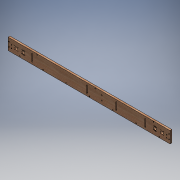
# Autodesk Inventor part: licht_150_top
Saved by Autodesk Inventor 2016 SP2 (Build 200236200, 236)
## iProperties
Created: 2018-01-11
Part Number: licht_150_top
Material: Spanplatte
Document SubType Name: Blech
Designer: schueler
Density: 1 g/cm^3
Sheet Metal Rule: Standard_mm
Appearance: Birke - natur- poliert
Mass: 2150.35 g
Surface Area: 3364.44 cm^2
Volume: 2150.35 cm^3
Author: schueler
Autodesk Inventor part; units mm, degrees
ref_plane "YZ Plane" through (0, 0, 0) normal (1, 0, 0) x (0, 1, 0)
ref_plane "XZ Plane" through (0, 0, 0) normal (0, 1, 0) x (-1, 0, 0)
ref_plane "XY Plane" through (0, 0, 0) normal (0, 0, 1) x (1, 0, 0)
sketch "Skizze1" plane through (0, 0, 0) normal (0, 1, 0) x (-1, 0, 0)
  line L0 (0, 0) -> (1392, 0)
  line L1 (1392, 0) -> (1392, -100)
  line L2 (1392, -100) -> (0, -100)
  line L3 (462, 0) -> (462, -100) construction
  line L4 (712, 0) -> (712, -100) construction
  line L5 (1292, 0) -> (1292, -100) construction
  line L6 (0, -92) -> (1392, -92) construction
  circle A0 centre (1292, -92) radius 1.5
  line L7 (1384, 0) -> (1384, -100) construction
  circle A1 centre (1384, -70) radius 1.5
  circle A2 centre (1384, -30) radius 1.5
  line L8 (1184.5, -137) -> (1184.5, -21) construction
  line L9 (1392, -8) -> (0, -8) construction
  circle A3 centre (1142, -8) radius 1.5
  line L10 (212, 0) -> (212, -100) construction
  line L11 (1092, 0) -> (1092, -100) construction
  line L12 (892, 0) -> (892, -100) construction
  line L13 (692, 0) -> (692, -100) construction
  line L14 (212, -16) -> (212, -16)
  line L15 (207, -21) -> (207, -79)
  line L16 (212, -84) -> (212, -84)
  line L17 (217, -79) -> (217, -21)
  arc A4 (217, -21) -> (212, -16) centre (212, -21) ccw
  arc A5 (212, -16) -> (207, -21) centre (212, -21) ccw
  arc A6 (207, -79) -> (212, -84) centre (212, -79) ccw
  arc A7 (212, -84) -> (217, -79) centre (212, -79) ccw
  circle A8 centre (1092, -92) radius 1.5
  circle A9 centre (892, -92) radius 1.5
  line L18 (92, 0) -> (92, -100) construction
  circle A10 centre (142, -8) radius 1.5
  circle A11 centre (92, -92) radius 1.5
  circle A12 centre (692, -92) radius 1.5
  circle A13 centre (642, -8) radius 1.5
  line L19 (292, 0) -> (292, -100) construction
  line L20 (492, 0) -> (492, -100) construction
  circle A14 centre (292, -92) radius 1.5
  circle A15 centre (492, -92) radius 1.5
  line L21 (462, -16) -> (462, -16)
  line L22 (457, -21) -> (457, -79)
  line L23 (467, -79) -> (467, -21)
  line L24 (1184.5, -84) -> (212, -84) construction
  line L25 (212, -16) -> (1184.5, -16) construction
  line L26 (1184.5, -21) -> (212, -21) construction
  line L27 (212, -79) -> (1184.5, -79) construction
  line L28 (712, -16) -> (712, -16)
  line L29 (707, -21) -> (707, -79)
  line L30 (712, -84) -> (712, -84)
  line L31 (717, -79) -> (717, -21)
  line L32 (1184.5, -16) -> (1184.5, -16)
  line L33 (1189.5, -21) -> (1189.5, -79)
  line L34 (1184.5, -84) -> (1184.5, -84)
  line L35 (1179.5, -79) -> (1179.5, -21)
  arc A16 (1189.5, -21) -> (1184.5, -16) centre (1184.5, -21) ccw
  arc A17 (1184.5, -16) -> (1179.5, -21) centre (1184.5, -21) ccw
  arc A18 (1179.5, -79) -> (1184.5, -84) centre (1184.5, -79) ccw
  arc A19 (1184.5, -84) -> (1189.5, -79) centre (1184.5, -79) ccw
  arc A20 (707, -79) -> (712, -84) centre (712, -79) ccw
  arc A21 (712, -84) -> (717, -79) centre (712, -79) ccw
  arc A22 (717, -21) -> (712, -16) centre (712, -21) ccw
  arc A23 (712, -16) -> (707, -21) centre (712, -21) ccw
  arc A24 (467, -21) -> (462, -16) centre (462, -21) ccw
  arc A25 (462, -16) -> (457, -21) centre (462, -21) ccw
  arc A26 (457, -79) -> (462, -84) centre (462, -79) ccw
  arc A27 (462, -84) -> (467, -79) centre (462, -79) ccw
  line L36 (0, -100) -> (0, 0)
  line L37 (8, 0) -> (8, -100) construction
  circle A28 centre (8, -30) radius 1.5
  circle A29 centre (8, -70) radius 1.5
  line L38 (8, -30) -> (1384, -30) construction
  line L39 (1384, -70) -> (8, -70) construction
  line L40 (1363, -100) -> (1363, 0) construction
  line L41 (29, 0) -> (29, -100) construction
  circle A30 centre (1363, -45) radius 1.5
  circle A31 centre (1363, -70) radius 1.5
  circle A32 centre (29, -70) radius 1.5
  circle A33 centre (29, -45) radius 1.5
  point P0 (1292, -8)
  point P1 (212, -16)
  point P2 (92, -8)
  point P3 (692, -8)
  point P4 (467, -16)
  point P5 (457, -84)
  point P6 (457, -16)
  point P7 (467, -84)
  point P8 (462, -16)
  point P9 (717, -16)
  point P10 (707, -84)
  point P11 (707, -16)
  point P12 (717, -84)
  point P13 (1179.5, -16)
  point P14 (1189.5, -84)
  point P15 (1189.5, -16)
  point P16 (1179.5, -84)
  dimension "d2" = 1392
  dimension "d3" = 100
  dimension "d8" = 100
  dimension "d15" = 8
  dimension "d18" = 3
  dimension "d20" = 8
  dimension "d25" = 3
  dimension "d26" = 3
  dimension "d44" = 30
  dimension "d45" = 30
  dimension "d59" = 3
  dimension "d60" = 200
  dimension "d61" = 200
  dimension "d62" = 200
  dimension "d66" = 10
  dimension "d67" = 5
  dimension "d72" = 3
  dimension "d74" = 3
  dimension "d78" = 250
  dimension "d80" = 3
  dimension "d81" = 3
  dimension "d82" = 3
  dimension "d83" = 3
  dimension "d92" = 200
  dimension "d93" = 200
  dimension "d95" = 3
  dimension "d96" = 3
  dimension "d102" = 10
  dimension "d103" = 16
  dimension "d104" = 16
  dimension "d107" = 10
  dimension "d108" = 10
  dimension "d111" = 5
  dimension "d112" = 5
  dimension "d113" = 5
  dimension "d114" = 250
  dimension "d115" = 500
  dimension "d120" = 8
  dimension "d122" = 250
  dimension "d158" = 207.5
  dimension "d159" = 680
  dimension "d160" = 200
  dimension "d161" = 500
  dimension "d163" = 8
  dimension "d164" = 3
  dimension "d165" = 3
  dimension "d175" = 29
  dimension "d176" = 29
  dimension "d177" = 3
  dimension "d178" = 3
  dimension "d179" = 15
  dimension "d180" = 3
  dimension "d181" = 3
  dimension "d182" = 15
  constraints: 78 end point, 62 point on line, 34 centre point, 32 point on circle, 31 tangent, 17 vertical, 12 equal radius, 9 parallel, 8 horizontal, 5 midpoint, 5 perpendicular, 1 collinear, 51 other
  measures "d2" distance of L1.end L36.start
  measures "d3" distance of L1.start L1.end
  measures "d8" distance of L1.start L5.start
  measures "d15" distance of L36.start point (0, -92)
  measures "d18" diameter of A0
  measures "d20" distance of L1.start L7.start
  measures "d25" diameter of A1
  measures "d26" diameter of A2
  measures "d59" diameter of A3
  measures "d60" distance between parallel lines of L11 L5
  measures "d61" distance between parallel lines of L12 L11
  measures "d62" distance between parallel lines of L13 L12
  measures "d66" distance between parallel lines of L15 L17
  measures "d67" radius of A4
  measures "d72" diameter of A8
  measures "d74" diameter of A9
  measures "d78" distance between parallel lines of L3 L10
  measures "d80" diameter of A10
  measures "d81" diameter of A11
  measures "d82" diameter of A12
  measures "d83" diameter of A13
  measures "d92" distance between parallel lines of L18 L19
  measures "d93" distance between parallel lines of L13 L20
  measures "d95" diameter of A14
  measures "d96" diameter of A15
  measures "d102" distance between parallel lines of L22 L23
  measures "d103" distance of the line from the sketch origin of L25
  measures "d107" distance between parallel lines of L35 L33
  measures "d108" distance between parallel lines of L29 L31
  measures "d111" radius of A16
  measures "d112" radius of A20
  measures "d113" radius of A24
  measures "d114" distance from line of L1 A3.centre
  measures "d115" distance of A3.centre A13.centre
  measures "d120" distance of the line from the sketch origin of L9
  measures "d122" distance between parallel lines of L3 L4
  measures "d158" distance between parallel lines of L1 L8
  measures "d159" distance between parallel lines of L1 L4
  measures "d160" distance between parallel lines of L19 L20
  measures "d161" distance of A10.centre A13.centre
  measures "d163" distance between parallel lines of L36 L37
  measures "d164" diameter of A28
  measures "d165" diameter of A29
  measures "d175" distance between parallel lines of L36 L41
  measures "d176" distance between parallel lines of L40 L1
  measures "d177" diameter of A30
  measures "d178" diameter of A31
  measures "d179" distance from line of L38 A30.centre
  measures "d180" diameter of A32
  measures "d181" diameter of A33
  measures "d182" distance from line of L38 A33.centre
extrude "Extrusion9" add sketch "Skizze1" along normal blind 16 contours L0 L1 L2 L36 | A28 | A29 | A30 | A31 | A32 | A33
sketch "Skizze4" plane through (0, 0, 0) normal (0, -1, 0) x (1, 0, 0)
  circle A0 centre (-92, -92) radius 1.5 projected
  circle A1 centre (-142, -8) radius 1.5 projected
  circle A2 centre (-292, -92) radius 1.5 projected
  circle A3 centre (-492, -92) radius 1.5 projected
  circle A4 centre (-642, -8) radius 1.5 projected
  circle A5 centre (-692, -92) radius 1.5 projected
  circle A6 centre (-892, -92) radius 1.5 projected
  circle A7 centre (-1092, -92) radius 1.5 projected
  circle A8 centre (-1292, -92) radius 1.5 projected
  circle A9 centre (-1142, -8) radius 1.5 projected
  circle A10 centre (-1384, -30) radius 1.5 projected
  circle A11 centre (-1384, -70) radius 1.5 projected
  line L0 (-1392, -100) -> (0, -100) construction
  line L1 (0, -100) -> (0, 0) construction
  line L2 (0, 0) -> (-1392, 0) construction
  line L3 (-1392, 0) -> (-1392, -100) construction
  line L4 (-1392, 0) -> (0, 0) construction
  line L5 (-587, 0) -> (-587, -100) construction
  arc A12 (-707, -21) -> (-717, -21) centre (-712, -21) ccw projected
  circle A13 centre (-8, -30) radius 1.5 projected
  circle A14 centre (-8, -70) radius 1.5 projected
  circle A15 centre (-1363, -70) radius 1.5 projected
  circle A16 centre (-1363, -45) radius 1.5 projected
  circle A17 centre (-29, -45) radius 1.5 projected
  circle A18 centre (-29, -70) radius 1.5 projected
  point P0 (-587, -30)
  point P1 (-587, -70)
  dimension "d133" = 30
  dimension "d134" = 30
  dimension "d162" = 125
  constraints: 10 end point, 6 coincident, 4 point on line, 2 parallel, 2 perpendicular, 1 horizontal
  measures "d133" distance of L5.start point (-587, -30)
  measures "d134" distance of L5.end point (-587, -70)
  measures "d162" distance from line of L5 A12.centre
hole "Bohrung3" at (-642, 0, -8) at (-692, 0, -92) at (-492, 0, -92) at (-292, 0, -92) at (-142, 0, -8) at (-92, 0, -92) at (-892, 0, -92) at (-1092, 0, -92) at (-1142, 0, -8) at (-1292, 0, -92) at (-1384, 0, -70) at (-1384, 0, -30) at (-587, 0, -70) at (-587, 0, -30) at (-8, 0, -30) at (-8, 0, -70) at (-1363, 0, -45) at (-1363, 0, -45) at (-1363, 0, -45) at (-1363, 0, -70) at (-1363, 0, -70) at (-1363, 0, -70) at (-29, 0, -70) at (-29, 0, -70) at (-29, 0, -70) at (-29, 0, -45) at (-29, 0, -45) at (-29, 0, -45) direction (0, 1, 0) diameter 3 end through all countersink diameter 8 countersink angle 90
sketch "Skizze5" plane through (0, 0, 0) normal (0, -1, 0) x (1, 0, 0)
  line L0 (-1392, 0) -> (-1392, -100) construction
  line L1 (-1392, -50) -> (-1322, -50) construction
  line L2 (-1336.6, -35.4) -> (-1307.4, -35.4) construction
  line L3 (-1307.4, -35.4) -> (-1307.4, -64.6) construction
  line L4 (-1307.4, -64.6) -> (-1336.6, -64.6) construction
  line L5 (-1336.6, -64.6) -> (-1336.6, -35.4) construction
  line L6 (-1322, 0) -> (-1322, -100) construction
  line L7 (0, -100) -> (-1392, -100) construction
  circle A0 centre (-1322, -50) radius 25.4 construction
  line L8 (-1276.6, -35.4) -> (-1247.4, -35.4) construction
  line L9 (-1247.4, -35.4) -> (-1247.4, -64.6) construction
  line L10 (-1247.4, -64.6) -> (-1276.6, -64.6) construction
  line L11 (-1276.6, -64.6) -> (-1276.6, -35.4) construction
  line L12 (-1392, 0) -> (0, 0) construction
  line L13 (-1262, 0) -> (-1262, -100) construction
  circle A1 centre (-1262, -50) radius 25.4 construction
  line L14 (-70, 0) -> (-70, -100) construction
  line L15 (-130, 0) -> (-130, -100) construction
  line L16 (0, -100) -> (0, 0) construction
  circle A2 centre (-70, -50) radius 25.4 construction
  circle A3 centre (-130, -50) radius 25.4 construction
  line L17 (-130, -50) -> (0, -50) construction
  line L18 (-144.6, -35.4) -> (-115.4, -35.4) construction
  line L19 (-115.4, -35.4) -> (-115.4, -64.6) construction
  line L20 (-115.4, -64.6) -> (-144.6, -64.6) construction
  line L21 (-144.6, -64.6) -> (-144.6, -35.4) construction
  line L22 (-84.6, -64.6) -> (-55.4, -64.6) construction
  line L23 (-55.4, -64.6) -> (-55.4, -35.4) construction
  line L24 (-55.4, -35.4) -> (-84.6, -35.4) construction
  line L25 (-84.6, -35.4) -> (-84.6, -64.6) construction
  point P0 (-1322, -35.4)
  point P1 (-1336.6, -50)
  point P2 (-1262, -35.4)
  point P3 (-115.4, -50)
  point P4 (-130, -35.4)
  point P5 (-70, -35.4)
  point P6 (-55.4, -50)
  dimension "d136" = 70
  dimension "d137" = 29.2
  dimension "d138" = 29.2
  dimension "d153" = 50.8
  dimension "d154" = 60
  dimension "d155" = 29.2
  dimension "d156" = 50.8
  dimension "d157" = 29.2
  dimension "d166" = 70
  dimension "d167" = 60
  dimension "d168" = 50.8
  dimension "d169" = 50.8
  dimension "d171" = 29.2
  dimension "d172" = 29.2
  dimension "d173" = 29.2
  dimension "d174" = 29.2
  constraints: 46 end point, 21 coincident, 14 point on line, 13 midpoint, 8 parallel, 7 perpendicular, 5 horizontal, 4 centre point, 2 vertical, 1 collinear
  measures "d136" distance between parallel lines of L0 L6
  measures "d137" distance of L3.end L4.end
  measures "d138" distance of L2.end L3.end
  measures "d153" diameter of A0
  measures "d154" distance between parallel lines of L13 L6
  measures "d155" distance of L8.start L8.end
  measures "d156" diameter of A1
  measures "d157" distance of L8.end L9.end
  measures "d166" distance between parallel lines of L16 L14
  measures "d167" distance between parallel lines of L15 L14
  measures "d168" diameter of A2
  measures "d169" diameter of A3
  measures "d171" distance of L19.end L20.end
  measures "d172" distance of L20.end L18.start
  measures "d173" distance of L22.start L22.end
  measures "d174" distance of L22.end L23.end
hole "Bohrung4" at (-1336.6, 0, -35.4) at (-1307.4, 0, -64.6) at (-1307.4, 0, -35.4) at (-1336.6, 0, -64.6) at (-1276.6, 0, -35.4) at (-1247.4, 0, -35.4) at (-1247.4, 0, -64.6) at (-1276.6, 0, -64.6) at (-144.6, 0, -35.4) at (-144.6, 0, -35.4) at (-115.4, 0, -35.4) at (-144.6, 0, -64.6) at (-144.6, 0, -64.6) at (-115.4, 0, -64.6) at (-115.4, 0, -64.6) at (-84.6, 0, -35.4) at (-84.6, 0, -35.4) at (-84.6, 0, -64.6) at (-55.4, 0, -35.4) at (-55.4, 0, -35.4) at (-55.4, 0, -64.6) direction (0, 1, 0) diameter 3 end through all
hole "Bohrung5" at (-1322, 0, -50) at (-1262, 0, -50) at (-130, 0, -50) at (-70, 0, -50) at (-70, 0, -50) direction (0, 1, 0) diameter 24 end through all
sketch "Skizze6" plane through (0, 0, 0) normal (0, -1, 0) x (1, 0, 0)
  circle A0 centre (-130, -50) radius 12 projected
  circle A1 centre (-1262, -50) radius 12 projected
  line L0 (-1269.5, -32.5) -> (-1254.5, -32.5)
  line L1 (-1254.5, -32.5) -> (-1254.5, -67.5)
  line L2 (-1254.5, -67.5) -> (-1269.5, -67.5)
  line L3 (-1269.5, -67.5) -> (-1269.5, -32.5)
  line L4 (-137.5, -32.5) -> (-122.5, -32.5)
  line L5 (-122.5, -32.5) -> (-122.5, -67.5)
  line L6 (-122.5, -67.5) -> (-137.5, -67.5)
  line L7 (-137.5, -67.5) -> (-137.5, -32.5)
  line L8 (-130, -50) -> (-122.5, -50) construction
  line L9 (-130, -50) -> (-130, -32.5) construction
  line L10 (-1262, -50) -> (-1254.5, -50) construction
  line L11 (-1262, -50) -> (-1262, -32.5) construction
  point P0 (0, 0)
  dimension "d183" = 15
  dimension "d184" = 35
  dimension "d185" = 15
  dimension "d186" = 35
  constraints: 24 end point, 5 perpendicular, 4 midpoint, 4 parallel, 2 horizontal, 1 point on line
  measures "d183" distance of L5.end L6.end
  measures "d184" distance of L4.end L5.end
  measures "d185" distance of L1.end L2.end
  measures "d186" distance of L0.end L1.end
extrude "Extrusion10" cut sketch "Skizze6" against normal blind 2 contours L5 A0 L7 | A0 L7 L4 L5 | L5 L6 L7 A0
extrude "Extrusion11" cut sketch "Skizze6" against normal blind 2 contours L1 A1 L3 | A1 L3 L0 L1 | L1 L2 L3 A1
equation "\"Biegeradius\" = Stärke"
equation "\"BreiteBiegungsfreistellung\" = Stärke"
equation "\"TiefeBiegungsfreistellung\" = 0.5 * Stärke"
equation "\"GrößeEckenfreistellung\" = 4 * Stärke"
equation "\"MinimalRest\" = 2 * Stärke"
equation "\"Übergangsradius\" = Biegeradius"
equation "\"JacobiRadiusGröße\" = Biegeradius"
equation "\"Abstandsgröße\" = Stärke"
equation "\"Stärke\" = 0.5"
